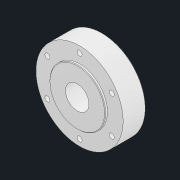
# Autodesk Inventor part: unit-base2
Saved by Autodesk Inventor 2021 (Build 250183000, 183)
## iProperties
Created: 2021-07-12
Part Number: unit-base2
Material: ABS プラスチック
Document SubType Name: Modeling
Designer: yuta0
Density: 1.06 g/cm^3
Appearance: 滑らか - 白
購入先: 印刷
在庫数: 0.0
Author: yuta0
Autodesk Inventor part; units mm, degrees
ref_plane "YZ Plane" through (0, 0, 0) normal (1, 0, 0) x (0, 1, 0)
ref_plane "XZ Plane" through (0, 0, 0) normal (0, 1, 0) x (-1, 0, 0)
ref_plane "XY Plane" through (0, 0, 0) normal (0, 0, 1) x (1, 0, 0)
sketch "スケッチ1" plane through (0, 0, 0) normal (1, 0, 0) x (0, 1, 0)
  line L0 (12.1, 0) -> (12.1, 5)
  line L1 (12.1, 5) -> (10.1, 5)
  line L2 (10.1, 5) -> (10.1, 22)
  line L3 (24, 20) -> (37.5, 20)
  line L4 (37.5, 20) -> (37.5, 0)
  line L5 (37.5, 0) -> (12.1, 0)
  line L6 (0, -4.4) -> (0, 26.4) projected
  line L7 (24, 20) -> (24, 22)
  line L8 (24, 22) -> (10.1, 22)
  point P0 (0, 0)
  dimension "d0" = 12.1
  dimension "d1" = 37.5
  dimension "d2" = 2
  dimension "d3" = 5
  dimension "d5" = 20
  dimension "d28" = 2
  dimension "d29" = 24
  constraints: 16 end point, 6 perpendicular, 2 vertical, 1 horizontal alignment
  measures "d0" distance from line of point (0, 0) L0
  measures "d1" distance from line of point (0, 0) L4
  measures "d2" distance of L0.end L1.end
  measures "d3" distance of L0.start L0.end
  measures "d5" distance of L3.end L4.end
  measures "d28" distance of L3.start L7.end
  measures "d29" distance between parallel lines of L6 L7
revolve "回転1" add sketch "スケッチ1" angle 360 about axis through (0, 0, -10) along (0, 0, 1)
chamfer "面取り1" distance 0.5 angle 45 1 edges at (0, -12.1, 0)
sketch "スケッチ2" plane through (0, 0, 20) normal (0, 0, 1) x (1, 0, 0)
  circle A0 centre (0, 0) radius 32
  point P0 (0, 32)
  point P1 (-27.7128, 16)
  point P2 (-27.7128, -16)
  point P3 (0, -32)
  point P4 (27.7128, -16)
  point P5 (27.7128, 16)
  dimension "d10" = 64
  dimension "d13" = 360
  constraints: 1 coincident, 1 vertical alignment, 9 other
hole "穴1" at (0, 32, 20) at (-27.7128, 16, 20) at (-27.7128, -16, 20) at (0, -32, 20) at (27.7128, -16, 20) at (27.7128, 16, 20) direction (0, 0, -1) diameter 4.3 end through all clearance for "Flat Head Machine Screw" size "M4" standard "Ansi Metric M Profile"
chamfer "面取り2" distance 1 angle 45 1 edges at (0, -37.5, 0)
chamfer "面取り3" distance 0.5 angle 45 1 edges at (0, -24, 22)
